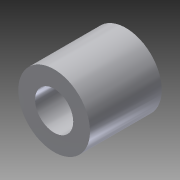
# Autodesk Inventor part: Wireless Mounting Board Spacer
Saved by Autodesk Inventor 2014 SP1 (Build 180222100, 222)
## iProperties
Created: 2013-10-26
Part Number: Wireless Mounting Board Spacer
Material: ABS Plastic
Document SubType Name: Modeling
Designer: Moses
Mass: 1.22268 g
Surface Area: 9.57924 cm^2
Volume: 1.15347 cm^3
Density: 1.06 g/cm^3
Appearance: Smooth - White
Author: Moses
Autodesk Inventor part; units mm, degrees
ref_plane "YZ Plane" through (0, 0, 0) normal (1, 0, 0) x (0, 1, 0)
ref_plane "XZ Plane" through (0, 0, 0) normal (0, 1, 0) x (-1, 0, 0)
ref_plane "XY Plane" through (0, 0, 0) normal (0, 0, 1) x (1, 0, 0)
sketch "Sketch1" plane through (0, 0, 0) normal (0, 0, 1) x (1, 0, 0)
  circle A0 centre (0, 0) radius 3.3782
  circle A1 centre (0, 0) radius 6.35
  dimension "d0" = 6.7564
  dimension "d1" = 12.7
  constraints: 2 centre point, 2 coincident
  measures "d0" diameter of A0
  measures "d1" diameter of A1
extrude "Extrusion1" add sketch "Sketch1" along normal blind 12.7
body "Solid1"
